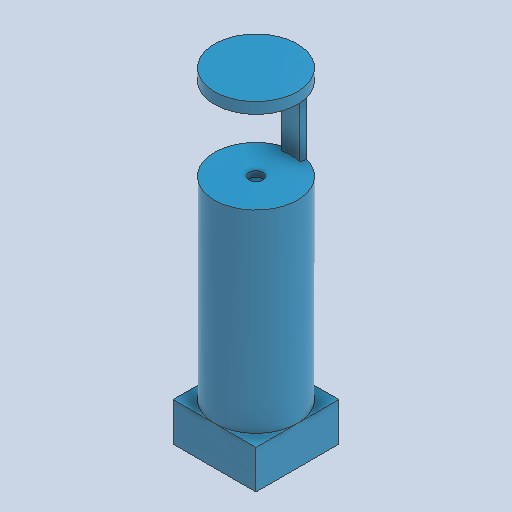
# Autodesk Inventor part: 1przegub
Saved by Autodesk Inventor 2022 (Build 260153000, 153)
## iProperties
Created: 2022-06-07
Part Number: 1przegub
Material: Ogólny
Document SubType Name: Sheet Metal
Designer: admin
Density: 1 g/cm^3
Sheet Metal Rule: Domyślny_mm
Appearance: Domyślna
Author: admin
Autodesk Inventor part; units mm, degrees
ref_plane "YZ Plane" through (0, 0, 0) normal (1, 0, 0) x (0, 1, 0)
ref_plane "XZ Plane" through (0, 0, 0) normal (0, 1, 0) x (-1, 0, 0)
ref_plane "XY Plane" through (0, 0, 0) normal (0, 0, 1) x (1, 0, 0)
sketch "Szkic1" plane through (0, 0, 0) normal (0, 1, 0) x (-1, 0, 0)
  line L0 (-75, 75) -> (75, 75)
  line L1 (75, 75) -> (75, -75)
  line L2 (75, -75) -> (-75, -75)
  line L3 (-75, -75) -> (-75, 75)
  line L4 (-75, 75) -> (75, -75) construction
  line L5 (75, 75) -> (-75, -75) construction
  point P0 (0, 0)
  dimension "d0" = 150
  dimension "d1" = 150
  constraints: 12 end point, 2 midpoint, 2 parallel, 1 horizontal, 1 perpendicular
  measures "d0" distance of L1.end L2.end
  measures "d1" distance of L0.end L1.end
extrude "Wyciągnięcie proste1" add sketch "Szkic1" along normal blind 70
sketch "Szkic2" plane through (0, 70, 0) normal (0, 1, 0) x (1, 0, 0)
  line L0 (-75, 75) -> (-75, -75) projected
  line L1 (75, 75) -> (-75, 75) projected
  line L2 (75, -75) -> (75, 75) projected
  line L3 (75, 75) -> (-75, 75) projected
  line L4 (-75, 75) -> (-75, -75) projected
  line L5 (-75, -75) -> (75, -75) projected
  line L6 (75, -75) -> (75, 75) projected
  circle A0 centre (0, 0) radius 75
  dimension "d4" = 150
  constraints: 1 centre point, 1 coincident
  measures "d4" diameter of A0
extrude "Wyciągnięcie proste2" add sketch "Szkic2" along normal blind 350 contours A0
sketch "Szkic3" plane through (0, 420, 0) normal (0, 1, 0) x (1, 0, 0)
  circle A0 centre (0, 0) radius 75 projected
  circle A1 centre (0, 0) radius 65
  line L0 (0, 0) -> (-19.4114, 72.4444)
  line L1 (0, 0) -> (19.4114, 72.4444)
  arc A2 (75, 0) -> (0, 75) centre (0, 0) ccw projected
  line L2 (0, 0) -> (0, 75)
  line L3 (75, 75) -> (-75, 75) projected
  point P0 (-16.8232, 62.7852)
  point P1 (16.8232, 62.7852)
  dimension "d7" = 130
  dimension "d8" = 15
  dimension "d9" = 15
  constraints: 6 end point, 2 line through centre, 2 point on circle, 1 centre point, 1 coincident, 1 perpendicular
  measures "d7" diameter of A1
  measures "d8" angle of L2 L1
  measures "d9" angle of L2 L0
extrude "Wyciągnięcie proste3" add sketch "Szkic3" along normal blind 150 contours L1 A1 L2 A0 | A0 L2 A1 L0
sketch "Szkic4" plane through (0, 570, 0) normal (0, 1, 0) x (1, 0, 0)
  circle A0 centre (0, 0) radius 75
  dimension "d12" = 150
  constraints: 1 centre point, 1 coincident
  measures "d12" diameter of A0
extrude "Wyciągnięcie proste4" add sketch "Szkic4" along normal blind 20
sketch "Szkic5" plane through (0, 420, 0) normal (0, 1, 0) x (1, 0, 0)
  circle A0 centre (0, 0) radius 12.5
  dimension "d15" = 25
  constraints: 1 centre point, 1 coincident
  measures "d15" diameter of A0
sketch "Szkic6" plane through (0, 570, 0) normal (0, -1, 0) x (1, 0, 0)
  circle A0 centre (0, 0) radius 12.5
  dimension "d18" = 25
  constraints: 1 centre point, 1 coincident
  measures "d18" diameter of A0
hole "Otwór1" at (0, 420, 0) direction (0, -1, 0) diameter 25 depth 10
hole "Otwór2" at (0, 570, 0) direction (0, 1, 0) diameter 25 depth 10
equation "\"PromieńGięcia\" = Grubość"
equation "\"SzerokośćGięciaPodcięcia\" = Grubość"
equation "\"GłębokośćGięciaPodcięcia\" = 0.5 * Grubość"
equation "\"RozmiarPodcięciaNarożnika\" = 4 * Grubość"
equation "\"MinimalnaPozostałość\" = 2 * Grubość"
equation "\"PromieńPrzejścia\" = PromieńGięcia"
equation "\"Rozmiar_promienia_Jacobiego\" = PromieńGięcia"
equation "\"Wielk_odstępu\" = Grubość"
equation "\"Grubość\" = 0.5"
